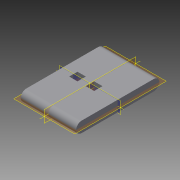
# Autodesk Inventor part: ChassisRechtsUntenKlappeSchluessel
Saved by Autodesk Inventor 2015 (Build 190159000, 159)
## iProperties
Created: 2018-12-06
Part Number: ChassisRechtsUntenKlappeSchluessel
Material: Generisch
Document SubType Name: Modeling
Designer: Boris
Density: 1 g/cm^3
Appearance: Vorgabe
Author: Boris
Autodesk Inventor part; units mm, degrees
sketch "Skizze1" plane through (0, 0, 0) normal (0, 0, 1) x (1, 0, 0)
  line L0 (-5, 7.5) -> (5, 7.5)
  line L1 (5, 7.5) -> (5, -7.5)
  line L2 (5, -7.5) -> (-5, -7.5)
  line L3 (-5, -7.5) -> (-5, 7.5)
  line L4 (-7, 0) -> (7, 0) projected
  line L5 (0, 10.5) -> (0, -10.5) projected
  point P0 (0, 0)
  dimension "d0" = 10
  dimension "d1" = 15
  constraints: 8 end point, 2 parallel, 1 horizontal, 1 perpendicular, 2 other
  measures "d0" distance of L1.end L2.end
  measures "d1" distance of L0.end L1.end
extrude "Extrusion1" add sketch "Skizze1" along normal mid plane 1.95
sketch "Skizze2" plane through (0, 0, 0.975) normal (0, 0, 1) x (1, 0, 0)
  line L0 (-5, 7.5) -> (-5, -7.5) projected
  line L1 (-3, -0.75) -> (-1.5, -0.75)
  line L2 (-1.5, -0.75) -> (-1.5, 0.75)
  line L3 (-1.5, 0.75) -> (-3, 0.75)
  line L4 (-3, 0.75) -> (-3, -0.75)
  line L5 (0, -0.75) -> (1.5, -0.75)
  line L6 (1.5, -0.75) -> (1.5, 0.75)
  line L7 (1.5, 0.75) -> (0, 0.75)
  line L8 (0, 0.75) -> (0, -0.75)
  line L9 (-7, 0) -> (7, 0) projected
  point P0 (0, 0)
  dimension "d4" = 1.5
  dimension "d5" = 2
  dimension "d6" = 1.5
  dimension "d7" = 1.5
  dimension "d8" = 1.5
  constraints: 16 end point, 4 parallel, 2 horizontal, 2 perpendicular, 2 point on line, 1 other
  measures "d4" distance of L3.end L1.start
  measures "d5" distance between parallel lines of L0 L4
  measures "d6" distance of L2.end L3.end
  measures "d7" distance between parallel lines of L8 L2
  measures "d8" distance of L6.end L7.end
extrude "Extrusion2" cut sketch "Skizze2" against normal blind 1.95
fillet "Rundung1" radius 1 4 edges at (0, 7.5, 0.975) (0, 7.5, -0.975) (0, -7.5, -0.975) (0, -7.5, 0.975)
